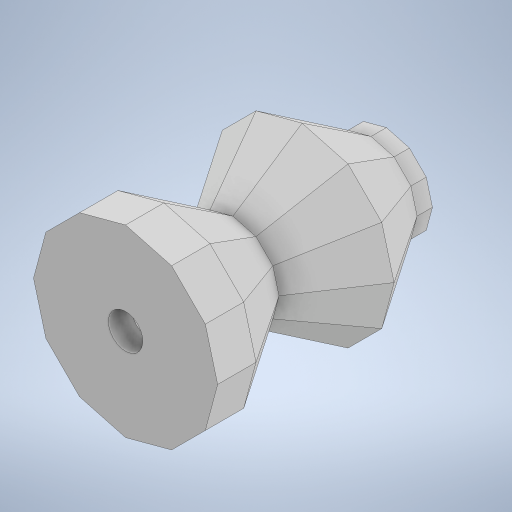
# Autodesk Inventor part: Test24.18.13
Saved by Autodesk Inventor 2023 (Build 270158000, 158)
## iProperties
Created: 2024-07-03
Part Number: Test24.18.13
Material: 일반
Document SubType Name: Modeling
Designer: ojs08
Density: 1 g/cm^3
Appearance: 기본값
Author: ojs08
Autodesk Inventor part; units mm, degrees
ref_plane "YZ Plane" through (0, 0, 0) normal (1, 0, 0) x (0, 1, 0)
ref_plane "XZ Plane" through (0, 0, 0) normal (0, 1, 0) x (-1, 0, 0)
sketch "스케치1" plane through (0, 0, 0) normal (0, 0, 1) x (1, 0, 0)
  line L0 (10.3923, 6) -> (12, 0)
  line L1 (12, 0) -> (10.3923, -6)
  line L2 (10.3923, -6) -> (6, -10.3923)
  line L3 (6, -10.3923) -> (0, -12)
  line L4 (0, -12) -> (-6, -10.3923)
  line L5 (-6, -10.3923) -> (-10.3923, -6)
  line L6 (-10.3923, -6) -> (-12, 0)
  line L7 (-12, 0) -> (-10.3923, 6)
  line L8 (-10.3923, 6) -> (-6, 10.3923)
  line L9 (-6, 10.3923) -> (0, 12)
  line L10 (0, 12) -> (6, 10.3923)
  line L11 (6, 10.3923) -> (10.3923, 6)
  line L12 (-16.8, 0) -> (16.8, 0) projected
  point P0 (0, 0)
  point P1 (0, 0)
  dimension "d0" = 24
  constraints: 24 end point, 1 coincident, 1 point on line, 25 other
  measures "d0" distance of L0.end L6.end
ref_plane "작업 평면1" through (0, 0, 9) normal (0, 0, 1) x (1, 0, 0)
sketch "스케치2" plane through (0, 0, 9) normal (0, 0, 1) x (1, 0, 0)
  line L0 (3, 5.1962) -> (5.1962, 3)
  line L1 (5.1962, 3) -> (6, 0)
  line L2 (6, 0) -> (5.1962, -3)
  line L3 (5.1962, -3) -> (3, -5.1962)
  line L4 (3, -5.1962) -> (0, -6)
  line L5 (0, -6) -> (-3, -5.1962)
  line L6 (-3, -5.1962) -> (-5.1962, -3)
  line L7 (-5.1962, -3) -> (-6, 0)
  line L8 (-6, 0) -> (-5.1962, 3)
  line L9 (-5.1962, 3) -> (-3, 5.1962)
  line L10 (-3, 5.1962) -> (0, 6)
  line L11 (0, 6) -> (3, 5.1962)
  line L12 (-16.8, 0) -> (16.8, 0) projected
  point P0 (0, 0)
  point P1 (0, 0)
  dimension "d2" = 12
  constraints: 24 end point, 1 coincident, 1 point on line, 25 other
  measures "d2" distance of L1.end L7.end
loft "로프트1" add profiles "스케치2", "스케치1"
mirror "미러1" about plane through (0, 0, 9) normal (0, 0, 1) of "로프트1"
mirror "미러2" about plane through (0, 0, 0) normal (0, 0, -1) of "로프트1"
sketch "스케치3" plane through (10.3923, 6, 18) normal (0, 0, 1) x (0.7071068, 0.7071068, 0)
  line L0 (0, 6.2117) -> (0, 0) projected
  line L1 (-3.1058, 11.5911) -> (0, 6.2117) projected
  line L2 (-8.4853, 14.6969) -> (-3.1058, 11.5911) projected
  line L3 (-14.6969, 14.6969) -> (-8.4853, 14.6969) projected
  line L4 (-20.0764, 11.5911) -> (-14.6969, 14.6969) projected
  line L5 (-23.1822, 6.2117) -> (-20.0764, 11.5911) projected
  line L6 (-23.1822, 0) -> (-23.1822, 6.2117) projected
  line L7 (-20.0764, -5.3795) -> (-23.1822, 0) projected
  line L8 (-14.6969, -8.4853) -> (-20.0764, -5.3795) projected
  line L9 (-8.4853, -8.4853) -> (-14.6969, -8.4853) projected
  line L10 (-3.1058, -5.3795) -> (-8.4853, -8.4853) projected
  line L11 (0, 0) -> (-3.1058, -5.3795) projected
  point P0 (-11.5911, 3.1058)
extrude "돌출1" add sketch "스케치3" along normal blind 3.3
shell "쉘5" thickness 1.3 removed faces 0 ; own thickness 2 on faces at (-10.2631, -2.75, -1.5) (-10.2631, 2.75, -1.5) (-7.5131, 7.5131, -1.5) (-7.5131, -7.5131, -1.5) (-2.75, -10.2631, -1.5) (2.75, -10.2631, -1.5) (7.5131, -7.5131, -1.5) (10.2631, -2.75, -1.5) (10.2631, 2.75, -1.5) (-2.75, 10.2631, -1.5) (2.75, 10.2631, -1.5) (7.5131, 7.5131, -1.5) (7.5131, 7.5131, 16.5) (10.2631, 2.75, 16.5) (10.2631, -2.75, 16.5) (7.5131, -7.5131, 16.5) (2.75, -10.2631, 16.5) (-2.75, -10.2631, 16.5) (-7.5131, -7.5131, 16.5) (-10.2631, -2.75, 16.5) (-10.2631, 2.75, 16.5) (-7.5131, 7.5131, 16.5) (-2.75, 10.2631, 16.5) (2.75, 10.2631, 16.5)
sketch "스케치16" plane through (10.3923, 6, 21.3) normal (0, 0, 1) x (0.7071068, -0.7071068, 0)
  line L0 (-11.5911, -3.1058) -> (-14.6969, -8.4853) projected
  line L1 (-14.6969, -8.4853) -> (-14.6969, -14.6969) projected
  line L2 (-14.6969, -14.6969) -> (-11.5911, -20.0764) projected
  line L3 (-11.5911, -20.0764) -> (-6.2117, -23.1822) projected
  line L4 (-6.2117, -23.1822) -> (0, -23.1822) projected
  line L5 (0, -23.1822) -> (5.3795, -20.0764) projected
  line L6 (5.3795, -20.0764) -> (8.4853, -14.6969) projected
  line L7 (8.4853, -14.6969) -> (8.4853, -8.4853) projected
  line L8 (8.4853, -8.4853) -> (5.3795, -3.1058) projected
  line L9 (5.3795, -3.1058) -> (0, 0) projected
  line L10 (0, 0) -> (-6.2117, 0) projected
  line L11 (-6.2117, 0) -> (-11.5911, -3.1058) projected
  point P0 (-3.1058, -11.5911)
extrude "돌출14" add sketch "스케치16" along normal blind 1.7
sketch "스케치17" plane through (10.3923, 6, 23) normal (0, 0, 1) x (0.7071068, 0.7071068, 0)
  circle A0 centre (-11.5911, 3.1058) radius 2.25
  dimension "d49" = 4.5
  constraints: 1 centre point, 1 coincident
  measures "d49" diameter of A0
extrude "돌출15" cut sketch "스케치17" against normal blind 3
sketch "스케치18" plane through (5.1962, 3, -9) normal (0, 0, -1) x (-0.7071068, -0.7071068, 0)
  line L0 (0, 3.1058) -> (0, 0) projected
  line L1 (0, 0) -> (1.5529, -2.6897) projected
  line L2 (1.5529, -2.6897) -> (4.2426, -4.2426) projected
  line L3 (4.2426, -4.2426) -> (7.3485, -4.2426) projected
  line L4 (7.3485, -4.2426) -> (10.0382, -2.6897) projected
  line L5 (10.0382, -2.6897) -> (11.5911, 0) projected
  line L6 (11.5911, 0) -> (11.5911, 3.1058) projected
  line L7 (11.5911, 3.1058) -> (10.0382, 5.7956) projected
  line L8 (10.0382, 5.7956) -> (7.3485, 7.3485) projected
  line L9 (7.3485, 7.3485) -> (4.2426, 7.3485) projected
  line L10 (4.2426, 7.3485) -> (1.5529, 5.7956) projected
  line L11 (1.5529, 5.7956) -> (0, 3.1058) projected
  point P0 (5.7956, 1.5529)
extrude "돌출16" add sketch "스케치18" along normal blind 2
